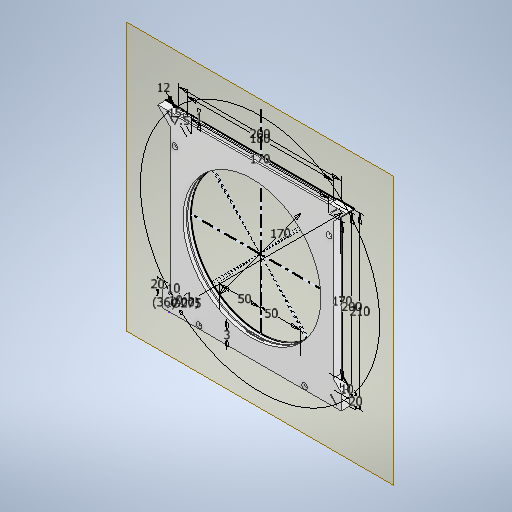
# Autodesk Inventor part: Target Holder and Sensor Plate
Saved by Autodesk Inventor 2025.1 (Build 291241000, 241)
## iProperties
Created: 2025-03-25
Part Number: Target Holder and Sensor Plate
Material: ABS Plastic
Document SubType Name: Modeling
Designer: maxwe
Density: 1.06 g/cm^3
Appearance: Smooth - White
Author: maxwe
## iProperties of the stored document Target Holder and Sensor Plate_3DPrint.ipt
Created: 2025-03-25
Part Number: Target Holder and Sensor Plate_3DPrint
Material: Generic
Document SubType Name: Modeling
Designer: maxwe
Density: 1 g/cm^3
Appearance: Default
Author: maxwe
Autodesk Inventor part; units mm, degrees
ref_plane "YZ Plane" through (0, 0, 0) normal (1, 0, 0) x (0, 1, 0)
ref_plane "XZ Plane" through (0, 0, 0) normal (0, 1, 0) x (-1, 0, 0)
ref_plane "XY Plane" through (0, 0, 0) normal (0, 0, 1) x (1, 0, 0)
ref_plane "Work Plane1" through (0, 0, 20) normal (0, 0, 1) x (1, 0, 0)
sketch "Sketch1" plane through (0, 0, 20) normal (0, 0, 1) x (1, 0, 0)
  line L0 (-90, -100) -> (90, -100)
  line L1 (90, -100) -> (90, 100)
  line L2 (90, 100) -> (-90, 100)
  line L3 (-90, 100) -> (-90, -100)
  line L4 (-90, -100) -> (90, 100) construction
  line L5 (90, -100) -> (-90, 100) construction
  line L6 (-100, -105) -> (100, -105)
  line L7 (100, -105) -> (100, 105)
  line L8 (100, 105) -> (-100, 105)
  line L9 (-100, 105) -> (-100, -105)
  line L10 (-100, -105) -> (100, 105) construction
  line L11 (100, -105) -> (-100, 105) construction
  line L12 (-85, -85) -> (85, -85)
  line L13 (85, -85) -> (85, 85)
  line L14 (85, 85) -> (-85, 85)
  line L15 (-85, 85) -> (-85, -85)
  line L16 (-85, -85) -> (85, 85) construction
  line L17 (85, -85) -> (-85, 85) construction
  line L18 (-85, 85) -> (-85, 105)
  line L19 (-90, 100) -> (-90, 105)
  line L20 (90, 100) -> (90, 105)
  line L21 (85, 85) -> (85, 105)
  line L22 (-50, -85) -> (-50, -108)
  line L23 (50, -85) -> (50, -108)
  line L24 (-100, -78) -> (-110, -88)
  line L25 (-110, -88) -> (-110, -108)
  line L26 (-110, -108) -> (110, -108)
  line L27 (110, -108) -> (110, -88)
  line L28 (110, -88) -> (100, -78)
  line L29 (-110, -88) -> (-100, -78)
  line L30 (-100, 89.3934) -> (-116.2886, 105.682)
  line L31 (-116.2886, 105.682) -> (-115.9706, 106)
  line L32 (-95.3934, 106) -> (-94.3934, 105)
  line L33 (0, 153.9952) -> (0, -108)
  line L34 (100, 89.3934) -> (116.2886, 105.682)
  line L35 (116.2886, 105.682) -> (115.9706, 106)
  line L36 (95.3934, 106) -> (94.3934, 105)
  line L37 (-103.9447, -104.6518) -> (-96.8736, -97.5807)
  line L38 (-97.5807, -96.8736) -> (-104.6518, -103.9447)
  arc A0 (-104.6518, -103.9447) -> (-103.9447, -104.6518) centre (-104.2983, -104.2983) ccw
  arc A1 (-96.8736, -97.5807) -> (-97.5807, -96.8736) centre (-97.2272, -97.2272) ccw
  line L39 (-100, 0) -> (100, 0)
  circle A2 centre (0, 0) radius 85
  line L40 (104.6518, -103.9447) -> (97.5807, -96.8736)
  arc A3 (97.5807, -96.8736) -> (96.8736, -97.5807) centre (97.2272, -97.2272) ccw
  line L41 (96.8736, -97.5807) -> (103.9447, -104.6518)
  arc A4 (103.9447, -104.6518) -> (104.6518, -103.9447) centre (104.2983, -104.2983) ccw
  line L42 (103.9447, 104.6518) -> (96.8736, 97.5807)
  arc A5 (96.8736, 97.5807) -> (97.5807, 96.8736) centre (97.2272, 97.2272) ccw
  line L43 (97.5807, 96.8736) -> (104.6518, 103.9447)
  arc A6 (104.6518, 103.9447) -> (103.9447, 104.6518) centre (104.2983, 104.2983) ccw
  line L44 (-104.6518, 103.9447) -> (-97.5807, 96.8736)
  arc A7 (-97.5807, 96.8736) -> (-96.8736, 97.5807) centre (-97.2272, 97.2272) ccw
  line L45 (-96.8736, 97.5807) -> (-103.9447, 104.6518)
  arc A8 (-103.9447, 104.6518) -> (-104.6518, 103.9447) centre (-104.2983, 104.2983) ccw
  line L46 (-95.3934, 106) -> (-115.9706, 106)
  line L47 (115.9706, 106) -> (95.3934, 106)
  point P0 (-50, -100)
  point P1 (-50, -105)
  point P2 (50, -100)
  point P3 (50, -105)
  point P4 (-110.9853, 110.9853)
  point P5 (-110.4295, -115.9509)
  point P6 (-99.3095, -105)
  point P7 (-100, -99.2929)
  point P8 (94.3934, 105)
  point P9 (100, 89.3934)
  point P10 (0, 85)
  point P11 (85, 0)
  point P12 (0, -85)
  point P13 (-85, 0)
  point P14 (-85, 100)
  point P15 (85, 100)
  point P16 (-90, -90.7071)
  point P17 (-90, -89.2929)
  point P18 (-100, -100.7071)
  dimension "d0" = 180
  dimension "d1" = 200
  dimension "d2" = 200
  dimension "d3" = 210
  dimension "d4" = 170
  dimension "d5" = 170
  dimension "d6" = 50
  dimension "d7" = 50
  dimension "d32" = 20
  dimension "d33" = 10
  dimension "d34" = 3
  dimension "d35" = 10
  dimension "d36" = 20
  dimension "d38" = 12
  dimension "d40" = 1
  dimension "d53" = 170
  dimension "d65" = 10
  dimension "d68" = 360
  dimension "d70" = 275
  dimension "d72" = 1
  dimension "d73" = 15
  dimension "d74" = 7.5
  constraints: 96 end point, 25 point on line, 16 perpendicular, 16 point on circle, 10 midpoint, 9 centre point, 9 parallel, 5 horizontal, 4 tangent, 3 symmetric about line, 2 vertical, 1 coincident, 1 horizontal alignment, 41 other
  measures "d0" distance of L2.end L1.end
  measures "d1" distance of L1.end L0.end
  measures "d2" distance of L8.end L7.end
  measures "d3" distance of L7.end L6.end
  measures "d4" distance of L14.end L13.end
  measures "d5" distance of L13.end L12.end
  measures "d6" distance from line of point (0, 0) L23
  measures "d7" distance from line of point (0, 0) L22
  measures "d32" distance of L24.end L25.end
  measures "d33" distance between parallel lines of L9 L25
  measures "d34" distance between parallel lines of L26 L6
  measures "d35" distance between parallel lines of L7 L27
  measures "d36" distance of L26.end L27.end
  measures "d38" distance from line of L31 L8.end
  measures "d40" diameter of A1
  measures "d53" diameter of A2
  measures "d65" distance of A0.centre A1.centre
  measures "d70" diameter of A1.centre point (0, 0)
  measures "d72" distance between parallel lines of L8 L46
  measures "d73" distance between parallel lines of L30 L32
  measures "d74" distance between parallel lines of L17 L30
extrude "Extrusion1" add sketch "Sketch1" along normal blind 10 contours L0 L22 L6 L9 L37 A1 L38 L39 L3 | L39 L9 L44 A7 L45 L8 L19 L3 | L22 L26 L25 L24 L9 L38 A0 L37 L6 | L0 L1 L39 L7 L40 A3 L41 L6 L23 | L30 L31 L46 L32 L8 L9 L45 A8 L44 | L6 L7 L41 A4 L40 L28 L27 L26 L23 | L1 L20 L8 L7 L42 A5 L43 L39 | L7 L43 A6 L42 L8 L36 L47 L35 L34
extrude "Extrusion2" add sketch "Sketch1" against normal blind 4.25 from surface at 10 contours L3 L39 L15 L12 L22 L0 | L22 L12 L33 L0 | L0 L33 L6 L22 | L3 L2 L18 L15 L39 | L33 L12 L23 L0 | L0 L23 L6 L33 | L6 L33 L26 L22 | L19 L8 L18 L2 | L23 L12 L13 L39 L1 L0 | L6 L23 L26 L33 | L13 L21 L2 L1 L39 | L21 L8 L20 L2
extrude "Extrusion3" add sketch "Sketch1" along normal blind 4.25 contours L3 L39 L15 L12 L22 L0 | L22 L12 L33 L0 | L0 L33 L6 L22 | L3 L2 L18 L15 L39 | L33 L12 L23 L0 | L0 L23 L6 L33 | L6 L33 L26 L22 | L19 L8 L18 L2 | L23 L12 L13 L39 L1 L0 | L6 L23 L26 L33 | L13 L21 L2 L1 L39 | L21 L8 L20 L2
chamfer "Chamfer3" distance 10 distance2 1.5 1 edges at (-90, 105, 25) measured on face at (-90, 104.5, 25)
chamfer "Chamfer4" distance 10 distance2 1.5 1 edges at (90, 105, 25) measured on face at (90, 104.5, 25)
chamfer "Chamfer5" distance 2 distance2 0.5 1 edges at (0, -85, 24.25) measured on face at (0, -85.5, 24.25)
chamfer "Chamfer6" distance 3 distance2 1 1 edges at (0, -85, 25.75) measured on face at (0, -85.5, 25.75)
sketch "Sketch2" plane through (0, 0, 30) normal (0, 0, 1) x (1, 0, 0)
  line L0 (-100, 89.3934) -> (-100, -78) projected
  line L1 (100, -78) -> (100, 89.3934) projected
  line L2 (-110, -108) -> (110, -108) projected
  line L3 (-110, -108) -> (110, -108) projected
  point P0 (0, 0)
  point P1 (-95, 72)
  point P2 (95, 72)
  point P3 (65, -104)
  point P4 (-65, -104)
  point P5 (-100, -99.2929)
  point P6 (-50, -108)
  dimension "d41" = 35
  dimension "d42" = 35
  dimension "d43" = 5
  dimension "d44" = 180
  dimension "d45" = 5
  dimension "d71" = 4
  constraints: 2 horizontal alignment
  measures "d41" distance from line of L0 point (-65, -104)
  measures "d42" distance from line of point (65, -104) L1
  measures "d43" distance from line of point (95, 72) L1
  measures "d44" distance from line of L2 point (95, 72)
  measures "d45" distance from line of L0 point (-95, 72)
  measures "d71" distance from line of L3 point (-65, -104)
hole "Hole1" at (-95, 72, 30) at (-65, -104, 30) at (65, -104, 30) at (95, 72, 30) direction (0, 0, -1) diameter 3.797 end through all countersink diameter 7.087 countersink angle 82 clearance for "Flat Head Machine Screw (82)" size "#6" standard "Ansi Unified Screw Threads"
extrude "Extrusion4" add sketch "Sketch1" along normal up to surface (4.25 mm away) contours L12 L15 A2 | L15 L14 A2 | A2 L13 L12 | L18 L8 L33 L2 | L2 L33 L14 L18 | L33 L2 L21 L14 | L14 L13 A2 | L33 L8 L21 L2
extrude "Extrusion5" add sketch "Sketch1" against normal up to surface (4.25 mm away) from surface at 10 contours L12 L15 A2 | L15 L14 A2 | A2 L13 L12 | L18 L8 L33 L2 | L2 L33 L14 L18 | L33 L2 L21 L14 | L14 L13 A2 | L33 L8 L21 L2
chamfer "Chamfer7" distance 2 distance2 6 1 edges at (0, 105, 24.25) measured on face at (0, 105, 23.75)
chamfer "Chamfer8" distance 2 distance2 6 1 edges at (0, 105, 25.75) measured on face at (0, 105, 26.25)
body "Solid1"
